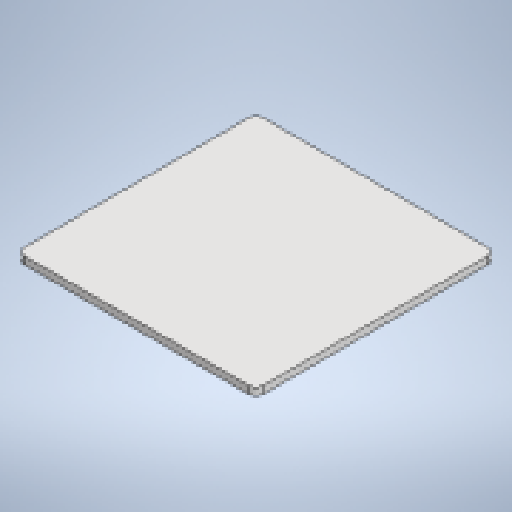
# Autodesk Inventor part: SLM 1424 FDS diam way cup
Saved by Autodesk Inventor 2025.3 (Build 293356030, 356C)
## iProperties
Created: 2025-06-24
Part Number: SLM 1424 FDS diam way cup
Material: Stainless Steel
Document SubType Name: Sheet Metal
Designer: admin
Mass: 93.5405 g
Surface Area: 123.051 cm^2
Volume: 11.6926 cm^3
Density: 8 g/cm^3
Flat Pattern Width: 6.4 cm
Flat Pattern Length: 6.4 cm
Flat Pattern Area: 40.96 cm^2
Sheet Metal Rule: AISI304 2mm Die16
Sheet Metal Width: 64,000 mm
Sheet Metal Length: 64,000 mm
Sheet Metal Area: 4096,000 mm^2
Appearance: Default
Author: user
Autodesk Inventor part; units mm, degrees
ref_plane "YZ Plane" through (0, 0, 0) normal (1, 0, 0) x (0, 1, 0)
ref_plane "XZ Plane" through (0, 0, 0) normal (0, 1, 0) x (-1, 0, 0)
ref_plane "XY Plane" through (0, 0, 0) normal (0, 0, 1) x (1, 0, 0)
sketch "Sketch1" plane through (0, 0, 0) normal (0, 0, 1) x (1, 0, 0)
  line L0 (-32, -32) -> (32, -32)
  line L1 (32, -32) -> (32, 32)
  line L2 (32, 32) -> (-32, 32)
  line L3 (-32, 32) -> (-32, -32)
  line L4 (-32, -32) -> (32, 32) construction
  line L5 (32, -32) -> (-32, 32) construction
  point P0 (0, 0)
  dimension "d154" = 64
  dimension "d155" = 64
  measures "d154" distance of L1.end L2.end
  measures "d155" distance of L0.end L1.end
extrude "Plate5" add sketch "Sketch1" along normal blind 2
fillet "Corner Round1" radius 2 4 edges at (32, 32, 1) (-32, -32, 1) (-32, 32, 1) (32, -32, 1)
sketch "Sketch11" plane through (-50.5, -22, -28) normal (1, 0, 0) x (0, 0, -1)
  line L0 (-25.25, 44) -> (-25.25, 0) construction
  line L1 (0, 0) -> (-25.25, 0) construction
  line L2 (0, 0) -> (0, 44) construction
  line L3 (0, 44) -> (-25.25, 44) construction
  circle A0 centre (-10, 22) radius 5.5
  point P0 (-28, 22)
  point P1 (0, 22)
  dimension "d192" = 11
  dimension "d193" = 10
  constraints: 1 centre point, 1 horizontal alignment, 1 midpoint
  measures "d192" diameter of A0
  measures "d193" distance from line of A0.centre L2
cut "Cut3" [suppressed]
feature "Corner Round3" [suppressed]
sketch "Sketch10" plane through (-34, 30, 2) normal (1, 0, 0) x (0, 1, 0)
  line L0 (-60, 0) -> (0, 0)
  line L1 (0, 0) -> (0, -30)
  line L2 (0, -30) -> (-60, -30)
  line L3 (-60, -30) -> (-60, 0)
  constraints: 8 end point
body "Solid3"
